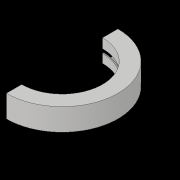
# Autodesk Inventor part: Outer_Shell_Bottom
Saved by Autodesk Inventor 2017 (Build 210142000, 142)
## iProperties
Created: 2017-01-10
Part Number: Outer_Shell_Bottom
Material: Generic
Document SubType Name: Modeling
Designer: David Kopala
Density: 1 g/cm^3
Appearance: Default
Author: David Kopala
Autodesk Inventor part; units mm, degrees
ref_plane "YZ Plane" through (0, 0, 0) normal (1, 0, 0) x (0, 1, 0)
ref_plane "XZ Plane" through (0, 0, 0) normal (0, 1, 0) x (-1, 0, 0)
ref_plane "XY Plane" through (0, 0, 0) normal (0, 0, 1) x (1, 0, 0)
sketch "Sketch1" plane through (0, 0, 0) normal (1, 0, 0) x (0, 1, 0)
  line L0 (0, 0) -> (50.8, 0)
  line L1 (0, 133.35) -> (0, 184.15)
  line L2 (0, 184.15) -> (73.025, 184.15)
  line L3 (73.025, 184.15) -> (73.025, 133.35)
  line L4 (69.85, 180.975) -> (3.175, 180.975)
  line L5 (3.175, 180.975) -> (3.175, 136.525)
  line L6 (69.85, 136.525) -> (69.85, 180.975)
  line L7 (29.2989, 148.3694) -> (29.2989, 120.4477)
  line L8 (41.9989, 148.9666) -> (41.9989, 122.6874)
  line L9 (0, 133.35) -> (29.2989, 133.35)
  line L10 (41.9989, 133.35) -> (73.025, 133.35)
  line L11 (3.175, 136.525) -> (29.2989, 136.525)
  line L12 (41.9989, 136.525) -> (69.85, 136.525)
  point P0 (3.175, 180.975)
  point P1 (69.85, 136.525)
  dimension "d0" = 50.8
  dimension "d3" = 50.8
  dimension "d4" = 73.025
  dimension "d5" = 3.175
  dimension "d6" = 3.175
  dimension "d7" = 3.175
  dimension "d8" = 3.175
  dimension "d9" = 3.175
  dimension "d11" = 3.175
  dimension "d13" = 26.1239
  dimension "d14" = 12.7
  dimension "d16" = 133.35
  dimension "d17" = 3.175
  dimension "d18" = 3.175
  constraints: 26 end point, 4 horizontal, 4 point on line, 3 parallel, 3 vertical, 2 perpendicular
  measures "d0" distance of L0.start L0.end
  measures "d3" distance of L1.start L1.end
  measures "d4" distance of L1.end L2.end
  measures "d5" distance from line of L3 L4.start
  measures "d6" distance from line of L2 L4.start
  measures "d7" distance from line of L2 point (3.175, 180.975)
  measures "d8" distance from line of L1 point (3.175, 180.975)
  measures "d9" distance from line of L1 L5.end
  measures "d11" distance from line of L3 point (69.85, 136.525)
  measures "d13" distance between parallel lines of L5 L7
  measures "d14" distance between parallel lines of L7 L8
  measures "d16" distance between parallel lines of L0 L9
  measures "d17" distance from line of L10 point (69.85, 136.525)
  measures "d18" distance from line of L9 L5.end
revolve "Revolution1" add sketch "Sketch1" angle 180 about axis through (0, 0, 0) along (0, 1, 0)
body "Solid1"
